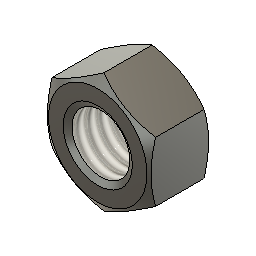
Modified Hotwire Files v11 (Autodesk Fusion 360 archive; units mm, degrees)
design "Hex Nut ANSI B18.2.2 - 3/8-16 Steel Grade 2H Plain"
description: Hex Nut ANSI B18.2.2 - 3/8-16
Autodesk Fusion 360 part; units mm, degrees
sketch "Sketch1" plane through (0, 0, 0) normal (0, 1, 0) x (1, 0, 0)
  line L0 (0, 0) -> (0, -8.3566)
  line L1 (-4.7625, 0) -> (-6.7926, 0)
  line L2 (-6.7926, 0) -> (-8.2584, -0.8463)
  line L3 (-8.2584, -0.8463) -> (-8.2584, -7.5103)
  line L4 (-8.2584, -7.5103) -> (-6.7926, -8.3566)
  line L5 (-6.7926, -8.3566) -> (-4.7625, -8.3566)
  line L6 (-4.7625, -8.3566) -> (-4.7625, 0)
  dimension "d121" = 9.525
  dimension "d122" = 30
  dimension "d123" = 30
  dimension "d125" = 13.5852
  dimension "d126" = 8.3566
  dimension "d127" = 13.5852
  dimension "d128" = 16.5167
  constraint vertical L0
  constraint coincident L0 L0.end
  constraint coincident origin L0
  constraint horizontal L1
  constraint perpendicular L1 L3
  constraint perpendicular L3 L5
  constraint perpendicular L5 L6
  constraint coincident L0.start L1
  constraint coincident L0.end L5
  constraint coincident L0.start origin
  measures "d122" angle of L1 L2
  measures "d123" angle of L4 L5
  measures "d126" distance of L1.start L5.end
revolve "Revolve1" add sketch "Sketch1" angle 360 about axis through (0, 0, 0) along (0, 0, 1)
sketch "Sketch8" plane through (0, 0, 8.3566) normal (0, 0, 1) x (1, 0, 0)
  line L0 (0, 0) -> (-14.3002, 0) construction
  line L1 (-7.1501, -4.1324) -> (-7.1501, 4.1324)
  circle A0 centre (0, 0) radius 4.7625
  circle A1 centre (0, 0) radius 8.2584
  dimension "d114" = 7.1501
  constraint horizontal L0
  constraint perpendicular L0 L1
  constraint midpoint L0 L1
  constraint coincident L0.start A0.centre
  constraint coincident L1.end A1
  measures "d114" distance of L0.start L1
extrude "Extrude5" cut sketch "Sketch8" against normal blind 8.3566 contours L1 A1 picked at (-7.3289, -1.0065)
pattern_circular "C-Pattern2" count 6 over 360 about axis through (0, 0, 1.75) along (0, 0, 1) of "Extrude5"
thread "Thread3" "ANSI Unified Screw Threads 0.375 3/8-16 UNC 2B" major diameter 9.525 minor diameter 7.9756 pitch 1.5875 angle 60 resizes the face on face at (-4.7566, 0.2374, 5.5711)
sketch "Sketch12" plane through (0, 0, 0) normal (0, 1, 0) x (1, 0, 0)
  line L0 (0, 0) -> (-4.7625, 0)
  line L1 (0, 0) -> (0, -8.3566)
  line L2 (0, -8.3566) -> (-4.7625, -8.3566)
  line L3 (-4.7625, -8.3566) -> (-2.2878, -6.9279)
  line L4 (-2.2878, -6.9279) -> (-2.2878, -8.3566)
  line L5 (-4.7625, 0) -> (-2.2878, -1.4287)
  line L6 (-2.2878, -1.4287) -> (-2.2878, 0)
  dimension "d164" = 30
  dimension "d165" = 30
  dimension "d166" = 4.7625
  dimension "d167" = 1.4288
  constraint coincident L0.start L1.start
  constraint horizontal L0
  constraint coincident L1.end L2.start
  constraint perpendicular L1 L2
  constraint coincident L2 L4.end
  constraint perpendicular L2 L4
  constraint coincident L0 L6.end
  constraint equal L4 L6
  constraint collinear L4 L6
  measures "d164" angle of L0 L5
  measures "d165" angle of L2 L3
  measures "d166" distance of L0.start L0.end
  measures "d167" distance of L5.end L6.end
revolve "Revolve3" cut sketch "Sketch12" angle 360 about axis through (0, 0, 1.75) along (0, 0, 1)
equation "d89 = -adsk_nheig"
equation "d114 = adsk_waflat / 2"
equation "adsk_chamang1 = 30.00 deg"
equation "adsk_chamang2 = 30.00 deg"
equation "d121 = adsk_nomdia"
equation "d122 = adsk_chamang1"
equation "d123 = adsk_chamang2"
equation "d125 = adsk_waflat * 0.95"
equation "d126 = adsk_nheig"
equation "d127 = adsk_waflat * 0.95"
equation "d128 = adsk_maxdia"
equation "adsk_nheig = 0.329 in"
equation "adsk_maxdia = 0.650265 in"
equation "adsk_nomdia = 0.375 in"
equation "adsk_waflat = 0.563 in"
equation "d162 = adsk_nheig"
equation "d166 = adsk_nomdia * 0.5"
equation "d167 = adsk_nomdia * 0.15"
